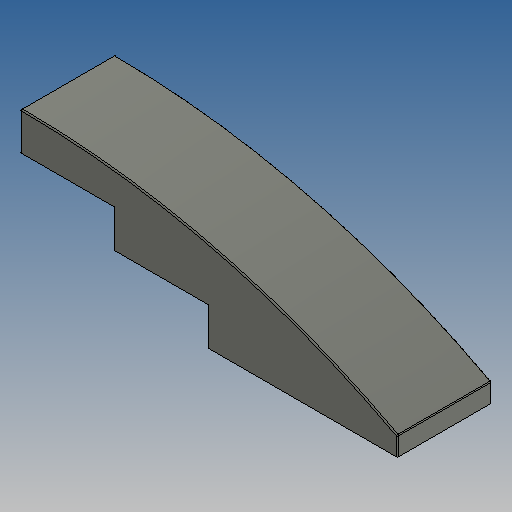
# Autodesk Inventor part: 11153-DkBluishGray
Saved by Autodesk Inventor 2025 (Build 290162010, 162A)
## iProperties
Created: 2014-06-03
Part Number: 11153-DkBluishGray
Material: ABS Plastic
Document SubType Name: Modeling
Designer: D. Kohfeld
Density: 1.06 g/cm^3
Appearance: DkBluishGray
Mass: 0.88337 g
Surface Area: 11.7156 cm^2
Volume: 0.833368 cm^3
Author: D. Kohfeld
Autodesk Inventor part; units mm, degrees
ref_plane "YZ Plane" through (0, 0, 0) normal (1, 0, 0) x (0, 1, 0)
ref_plane "XZ Plane" through (0, 0, 0) normal (0, 1, 0) x (-1, 0, 0)
ref_plane "XY Plane" through (0, 0, 0) normal (0, 0, 1) x (1, 0, 0)
sketch "Sketch2" plane through (0, 0, 0) normal (0, 1, 0) x (-1, 0, 0)
  line L0 (-16, 4) -> (16, 4)
  line L1 (16, 4) -> (16, -4)
  line L2 (16, -4) -> (-16, -4)
  line L3 (-16, -4) -> (-16, 4)
  point P0 (0, 0)
  point P1 (0, 4)
  point P2 (-16, 0)
  dimension "d0" = 32
  dimension "d1" = 8
  constraints: 8 end point, 2 midpoint, 2 parallel, 1 horizontal, 1 horizontal alignment, 1 perpendicular, 1 vertical alignment
  measures "d0" distance of L1.end L2.end
  measures "d1" distance of L2.end L0.start
extrude "Extrusion1" add sketch "Sketch2" along normal blind 9.6
sketch "Sketch10" plane through (0, 0, 0) normal (0, 0, 1) x (1, 0, 0)
  line L0 (-16, 9.6) -> (16, 9.6) projected
  line L1 (-16, 0) -> (-16, 9.6) projected
  arc A0 (16, 1.6) -> (-16, 9.6) centre (-16, -58.4) ccw
  line L2 (16, 1.6) -> (16, 9.6)
  line L3 (-16, 0) -> (16, 0) projected
  line L4 (14.4, 0) -> (14.4, 1.6)
  line L5 (14.4, 1.6) -> (12.4422, 1.6)
  line L6 (-8, 3.2) -> (-8, 7.5163)
  line L7 (-6.4, 7.3024) -> (-6.4, 3.2)
  arc A1 (12.4422, 1.6) -> (-6.4, 7.3024) centre (-16, -58.4) ccw
  arc A2 (-8, 7.5163) -> (-14.4, 7.9807) centre (-16, -58.4) ccw
  line L8 (-14.4, 7.9807) -> (-14.4, 6.4)
  line L9 (1.6, 5.625) -> (1.6, 0)
  line L10 (0, 6.0435) -> (0, 0)
  line L11 (0, 3.2) -> (-6.4, 3.2)
  line L12 (-8, 6.4) -> (-14.4, 6.4)
  line L13 (-14.4, 6.4) -> (-16, 6.4)
  line L14 (16, 0) -> (16, 9.6) projected
  line L15 (1.6, 0) -> (14.4, 0)
  line L16 (0, 0) -> (-16, 0)
  line L17 (-16, 0) -> (-16, 6.4)
  line L18 (-6.4, 3.2) -> (-8, 3.2)
  dimension "d100" = 1.6
  dimension "d104" = 1.6
  dimension "d105" = 1.6
  dimension "d107" = 1.6
  dimension "d108" = 1.6
  dimension "d113" = 6.4
  dimension "d114" = 3.2
  dimension "d115" = 16
  dimension "d116" = 1.6
  constraints: 30 end point, 8 perpendicular, 8 point on circle, 5 point on line, 4 parallel, 3 centre point, 3 collinear, 2 concentric, 1 midpoint, 1 tangent
  measures "d100" distance from line of L2.start L3
  measures "d104" distance from line of L4 L3.end
  measures "d105" distance between parallel lines of L5 L3
  measures "d107" radial gap between concentric circles of A0 A2
  measures "d108" distance between parallel lines of L1 L8
  measures "d113" distance between parallel lines of L13 L3
  measures "d114" distance between parallel lines of L11 L3
  measures "d115" distance between parallel lines of L14 L10
  measures "d116" distance between parallel lines of L10 L9
extrude "Extrusion7" cut sketch "Sketch10" along normal through all both and the other way through all contours L0 L2 A0 | L13 L12 L6 L18 L11 L10 L3 L1
extrude "Extrusion8" cut sketch "Sketch10" along normal mid plane 4.8 contours L8 A2 L6 L12 | L3 L9 A1 L5 L4 | L11 L7 A1 L10
sketch "Sketch3" plane through (0, 0, 0) normal (0, -1, 0) x (1, 0, 0)
  circle A0 centre (12, 0) radius 2.4 construction
  line L0 (14.4, -2.4) -> (1.6, -2.4) projected
  line L1 (1.6, -2.4) -> (1.6, 2.4) projected
  line L2 (1.6, 2.4) -> (14.4, 2.4) projected
  line L3 (14.4, 2.4) -> (14.4, -2.4) projected
  line L4 (16, 4) -> (0, 4) projected
  circle A1 centre (4, 0) radius 2.4 construction
  line L5 (5.3971, 2.4) -> (5.3971, 1.9971)
  line L6 (5.3971, 1.9971) -> (5.9971, 1.3971)
  line L7 (5.9971, 1.3971) -> (6.5971, 1.9971)
  line L8 (6.5971, 1.9971) -> (6.5971, 2.4)
  line L9 (10.6029, 2.4) -> (10.6029, 1.9971)
  line L10 (10.6029, 1.9971) -> (10.0029, 1.3971)
  line L11 (10.0029, 1.3971) -> (9.4029, 1.9971)
  line L12 (9.4029, 1.9971) -> (9.4029, 2.4)
  line L13 (5.3971, -2.4) -> (5.3971, -1.9971)
  line L14 (5.3971, -1.9971) -> (5.9971, -1.3971)
  line L15 (5.9971, -1.3971) -> (6.5971, -1.9971)
  line L16 (6.5971, -1.9971) -> (6.5971, -2.4)
  line L17 (9.4029, -2.4) -> (9.4029, -1.9971)
  line L18 (9.4029, -1.9971) -> (10.0029, -1.3971)
  line L19 (10.0029, -1.3971) -> (10.6029, -1.9971)
  line L20 (10.6029, -1.9971) -> (10.6029, -2.4)
  line L21 (5.6971, 1.6971) -> (4, 0) construction
  dimension "d97" = 4.8
  dimension "d118" = 1.2
  constraints: 34 end point, 12 perpendicular, 11 equal length, 9 tangent, 8 point on line, 4 parallel, 2 centre point, 1 coincident, 1 midpoint
  measures "d97" diameter of A0
  measures "d118" distance between parallel lines of L8 L5
extrude "Extrusion2" add sketch "Sketch3" against normal up to next contours L0 L17 L18 L19 L20 | L9 L10 L11 L12 L2 | L0 L13 L14 L15 L16 | L8 L7 L6 L5 L2
sketch "Sketch11" plane through (-8, 3.2, 4) normal (0, -1, 0) x (1, 0, 0)
  line L0 (1.6, -1.6) -> (8, -1.6) projected
  line L1 (8, -1.6) -> (8, 0) projected
  line L2 (8, -6.4) -> (1.6, -6.4) projected
  line L3 (1.6, -6.4) -> (1.6, -1.6) projected
  circle A0 centre (4, -4) radius 2.4 construction
  line L4 (8, -3.4) -> (6.4, -3.4)
  line L5 (6.4, -3.4) -> (6.4, -4.6)
  line L6 (6.4, -4.6) -> (8, -4.6)
  line L7 (8, -3.4) -> (8, -4.6)
  point P0 (8, -4)
  point P1 (6.4, -4)
  dimension "d119" = 1.2
  constraints: 8 end point, 4 tangent, 3 perpendicular, 1 centre point, 1 collinear, 1 horizontal alignment, 1 midpoint, 1 parallel, 1 vertical alignment
  measures "d119" distance of L4.end L5.end
extrude "Extrusion9" add sketch "Sketch11" against normal up to next
sketch "Sketch12" plane through (-16, 6.4, 4) normal (0, -1, 0) x (1, 0, 0)
  line L0 (1.6, -1.6) -> (8, -1.6) projected
  line L1 (8, -6.4) -> (1.6, -6.4) projected
  line L2 (1.6, -6.4) -> (1.6, -1.6) projected
  line L3 (8, -3.4) -> (6.4, -3.4)
  line L4 (6.4, -3.4) -> (6.4, -4.6)
  line L5 (6.4, -4.6) -> (8, -4.6)
  line L6 (8, -4.6) -> (8, -3.4)
  circle A0 centre (4, -4) radius 2.4 construction
  point P0 (16, -4)
  point P1 (6.4, -4)
  dimension "d122" = 1.2
  constraints: 8 end point, 4 tangent, 2 parallel, 1 centre point, 1 horizontal, 1 horizontal alignment, 1 midpoint, 1 perpendicular, 1 vertical alignment
  measures "d122" distance between parallel lines of L3 L5
extrude "Extrusion10" add sketch "Sketch12" against normal up to next
fillet "Fillet1" radius 0.1 8 edges at (-16, 8, 4) (-16, 9.6, 0) (16, 0.8, 4) (16, 0.8, -4) (-16, 8, -4) (0.4924, 7.5697, 4) (0.4924, 7.5697, -4) (16, 1.6, 0)
equation "\"d4\" = lh"
equation "\"d100\" = wall"
equation "\"d104\" = wall"
equation "\"d105\" = 0.333333 * lh - topthk"
equation "\"d107\" = topthk"
equation "\"d108\" = d104"
equation "\"d113\" = 0.666667 * lh"
equation "\"d114\" = 0.333333 * lh"
equation "\"d115\" = 2 * lu"
equation "\"d116\" = wall"
equation "\"d109\" = lu - 2 * wall"
equation "\"d97\" = kd"
equation "\"d22\" = lf"
equation "\"d103\" = d102"
equation "\"lh\" = 9.6"
equation "\"wall\" = 1.6"
equation "\"topthk\" = 1.6"
equation "\"lu\" = 8"
equation "\"kd\" = 4.8"
equation "\"lf\" = 0.1"
equation "\"d102\" = 1.6"
body "Solid1"
